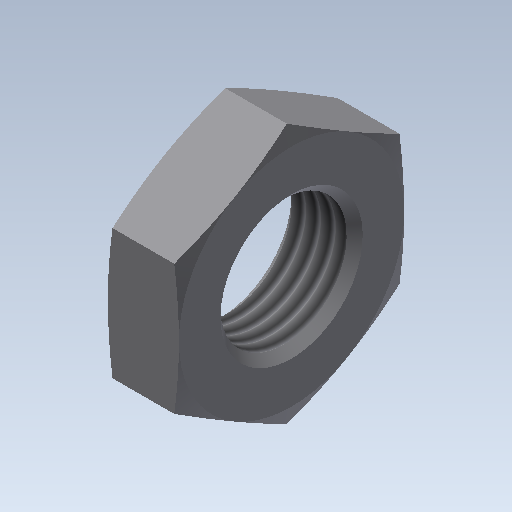
# Autodesk Inventor part: RM/8010_N
Saved by Autodesk Inventor 2020.5 (Build 245400000, 400)
## iProperties
Created: 2018-09-27
Part Number: RM/8010_N
Material: Generic
Catalog Web Link: www.cadenas.de
Description: Series RM/8000/M NUT-ISO Cylinder
Vendor: IMI
Document SubType Name: Modeling
Designer: psadmin
Manufacturer: IMI
Mass: 1.31875 g
Surface Area: 10.0176 cm^2
Volume: 1.31875 cm^3
Density: 1 g/cm^3
Appearance: PSOLRGB-192-192-192
Category: PARTsolutions
Company: IMI
PSOL_IDENT_0: {$CADENAS_DATA\23d-libs\imi_precision\1_actuators\1_roundline_cylinders\parts\series_rm_8000_m_nut.p
PSOL_IDENT_1: rj},172 {VTYP=3D},{NB=RM/8010_N},{LINA=RM/8010_N},{NN=Series RM/8000/M NUT},{DATE=04.09.2018 05:58:3
PSOL_IDENT_2: 0},{GEOMDATE=13.09.2016 06:18:00},{VERSION=},{LINEID=10},{WBVAR=},{WBNUMERIC=}  {NB=RM/8010_N},{LINA=
PSOL_IDENT_3: RM/8010_N},{KT=DUMMY},{CNSORDERNO=RM/8010},{BS=010},{BSX=10},{BE=M12x1.25},{BEX=12.000},{BEP=1.250},
PSOL_IDENT_4: {KV=19},{KW=6}
NN: Series RM/8000/M NUT
NT: ISO Cylinder
NB: RM/8010_N
NBSYN: $CNSORDERNO._N
LINA: RM/8010_N
CNSORDERNO: RM/8010
BS: 010
BSX: 10
BE: M12x1.25
KV: 19
KW: 6
SUPPLIER: IMI
ARTICLENO: RM/8010_N
BOMINFO: RM/8010_N
CREATOR: CADENAS GmbH
Title: RM/8010_N
Author: Cadenas PARTsolutions
Comments: ISO Cylinder
Autodesk Inventor part; units mm, degrees
sketch "Sketch_1" plane through (0, 0, 0) normal (0, 0, 1) x (1, 0, 0)
  line L0 (3, 0) -> (-3, 0)
  line L1 (-3, 6) -> (-2.3235, 5.3235)
  line L2 (-2.3235, 5.3235) -> (2.3235, 5.3235)
  line L3 (2.3235, 5.3235) -> (3, 6)
  line L4 (3, 6) -> (3, 9.5)
  line L5 (3, 9.5) -> (1.4471, 15.2956)
  line L6 (1.4471, 15.2956) -> (-1.4471, 15.2956)
  line L7 (-1.4471, 15.2956) -> (-3, 9.5)
  line L8 (-3, 9.5) -> (-3, 6)
  constraints: 18 end point
revolve "Revolution1" add sketch "Sketch_1" angle 360 about axis through (3, 0, 0) along (1, 0, 0)
thread "Thread1" size "M12x1.25" class "6H" standard "ISO Metric profile" full length
sketch "Sketch_2" plane through (0, 0, 0) normal (1, 0, 0) x (0, 1, 0)
  line L0 (-38, 38) -> (-38, -38)
  line L1 (-38, -38) -> (38, -38)
  line L2 (38, -38) -> (38, 38)
  line L3 (38, 38) -> (-38, 38)
  line L4 (-5.4848, 9.5) -> (-10.9697, 0)
  line L5 (-10.9697, 0) -> (-5.4848, -9.5)
  line L6 (-5.4848, -9.5) -> (5.4848, -9.5)
  line L7 (5.4848, -9.5) -> (10.9697, 0)
  line L8 (10.9697, 0) -> (5.4848, 9.5)
  line L9 (5.4848, 9.5) -> (-5.4848, 9.5)
  constraints: 20 end point
extrude "Extrusion1" cut sketch "Sketch_2" along normal mid plane 6
ref_plane "NUT_XY" through (-3, 0, 0) normal (1, 0, 0) x (0, 0, -1)
ref_plane "NUT_YZ" through (-3, 0, 0) normal (0, 0, -1) x (0, 1, 0)
ref_plane "NUT_ZX" through (-3, 0, 0) normal (0, 1, 0) x (1, 0, 0)
ref_plane "dim_kv1_XY" through (0, 5.4848, 9.5) normal (1, 0, 0) x (0, 0, -1)
ref_plane "dim_kv1_YZ" through (0, 5.4848, 9.5) normal (0, 0, -1) x (0, 1, 0)
ref_plane "dim_kv1_ZX" through (0, 5.4848, 9.5) normal (0, 1, 0) x (1, 0, 0)
ref_plane "dim_kv2_XY" through (0, 5.4848, -9.5) normal (1, 0, 0) x (0, 0, -1)
ref_plane "dim_kv2_YZ" through (0, 5.4848, -9.5) normal (0, 0, -1) x (0, 1, 0)
ref_plane "dim_kv2_ZX" through (0, 5.4848, -9.5) normal (0, 1, 0) x (1, 0, 0)
ref_plane "dim_kw1_XY" through (-3, 9.5, 0) normal (0, 0, 1) x (1, 0, 0)
ref_plane "dim_kw1_YZ" through (-3, 9.5, 0) normal (1, 0, 0) x (0, 1, 0)
ref_plane "dim_kw1_ZX" through (-3, 9.5, 0) normal (0, 1, 0) x (0, 0, 1)
ref_plane "dim_kw2_XY" through (3, 9.5, 0) normal (0, 0, 1) x (1, 0, 0)
ref_plane "dim_kw2_YZ" through (3, 9.5, 0) normal (1, 0, 0) x (0, 1, 0)
ref_plane "dim_kw2_ZX" through (3, 9.5, 0) normal (0, 1, 0) x (0, 0, 1)
body "Solid1"
